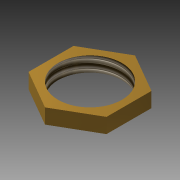
# Autodesk Inventor part: KeySwitchNut
Saved by Autodesk Inventor 2016 (Build 200138000, 138)
## iProperties
Created: 2014-09-27
Part Number: KeySwitchNut
Material: Generic
Document SubType Name: Modeling
Designer: Jack
Density: 1 g/cm^3
Appearance: Brass - Satin
Mass: 0.691687 g
Surface Area: 8.86962 cm^2
Volume: 0.691687 cm^3
Author: Jack
Autodesk Inventor part; units mm, degrees
ref_plane "YZ Plane" through (0, 0, 0) normal (1, 0, 0) x (0, 1, 0)
ref_plane "XZ Plane" through (0, 0, 0) normal (0, 1, 0) x (-1, 0, 0)
ref_plane "XY Plane" through (0, 0, 0) normal (0, 0, 1) x (1, 0, 0)
sketch "Sketch1" plane through (0, 0, 0) normal (0, 0, 1) x (1, 0, 0)
  line L0 (0, 12.7017) -> (11, 6.3509)
  line L1 (11, 6.3509) -> (11, -6.3509)
  line L2 (11, -6.3509) -> (0, -12.7017)
  line L3 (0, -12.7017) -> (-11, -6.3509)
  line L4 (-11, -6.3509) -> (-11, 6.3509)
  line L5 (-11, 6.3509) -> (0, 12.7017)
  circle A0 centre (0, 0) radius 9
  dimension "d0" = 22
  dimension "d1" = 18
  constraints: 12 end point, 2 coincident, 1 centre point, 1 vertical, 13 other
  measures "d0" distance between parallel lines of L1 L4
  measures "d1" diameter of A0
extrude "Extrusion1" add sketch "Sketch1" along normal blind 4.2
thread "Thread1" size "M18x2.5" class "6H" standard "ANSI Metric M Profile" full length
body "Solid1"
